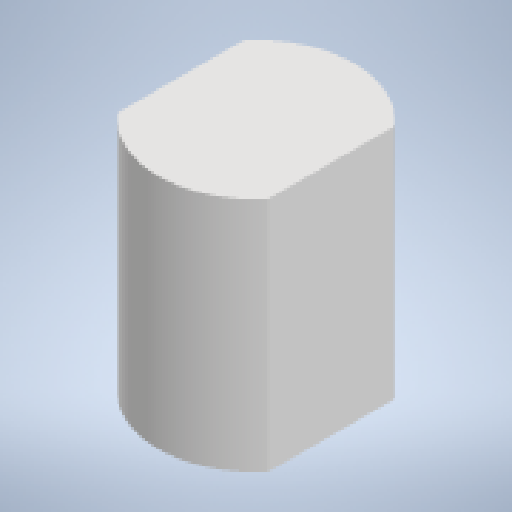
# Autodesk Inventor part: moteurG6V2
Saved by Autodesk Inventor 2025.2 (Build 292293000, 293)
## iProperties
Created: 2025-02-21
Part Number: moteurG6V2
Material: Générique
Document SubType Name: Modeling
Designer: antoi
Density: 1 g/cm^3
Appearance: Par défaut
Author: antoi
Autodesk Inventor part; units mm, degrees
ref_plane "YZ Plane" through (0, 0, 0) normal (1, 0, 0) x (0, 1, 0)
ref_plane "XZ Plane" through (0, 0, 0) normal (0, 1, 0) x (-1, 0, 0)
ref_plane "XY Plane" through (0, 0, 0) normal (0, 0, 1) x (1, 0, 0)
sketch "Esquisse1" plane through (0, 0, 0) normal (0, 1, 0) x (-1, 0, 0)
  line L0 (5.9, -4.9477) -> (5.9, 4.9477)
  line L1 (-5.9, -4.9477) -> (-5.9, 4.9477)
  arc A0 (5.9, 4.9477) -> (-5.9, 4.9477) centre (0, 0) ccw
  arc A1 (-5.9, -4.9477) -> (5.9, -4.9477) centre (0, 0) ccw
  constraints: 4 end point, 4 point on circle, 2 centre point, 1 coincident
extrude "Extrusion1" add sketch "Esquisse1" along normal blind 18.6
